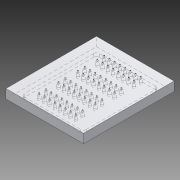
# Autodesk Inventor part: UNLHEP-14-01-P-001_ModuleChuck
Saved by Autodesk Inventor 2013 (Build 170138000, 138)
## iProperties
Created: 2014-01-06
Part Number: UNLHEP-14-01-P-001_ModuleChuck
Material: Aluminium 6061
Document SubType Name: Modeling
Designer: Frank Meier
Density: 2.71 g/cm^3
Project: UNL Pixel Phase I
Description: ModuleChuck
Mass: 472.689 g
Surface Area: 484.697 cm^2
Volume: 174.424 cm^3
Author: Frank Meier
Revision Number: 00
Title: Bonder Chuck
Autodesk Inventor part; units mm, degrees
ref_plane "YZ Plane" through (0, 0, 0) normal (1, 0, 0) x (0, 1, 0)
ref_plane "XZ Plane" through (0, 0, 0) normal (0, 1, 0) x (-1, 0, 0)
ref_plane "XY Plane" through (0, 0, 0) normal (0, 0, 1) x (1, 0, 0)
sketch "Skizze1" plane through (0, 0, 0) normal (0, 0, 1) x (1, 0, 0)
  line L0 (60, -70) -> (-60, -70)
  line L1 (-60, -70) -> (-60, 70)
  line L2 (-60, 70) -> (60, 70)
  line L3 (60, 70) -> (60, -70)
  line L4 (60, -70) -> (-60, 70) construction
  line L5 (-60, -70) -> (60, 70) construction
  point P0 (0, 0)
  dimension "d0" = 120
  dimension "d3" = 140
  constraints: 12 end point, 2 midpoint, 2 parallel, 1 horizontal, 1 perpendicular
  measures "d0" distance of L1.end L2.end
  measures "d3" distance of L0.end L1.end
extrude "Extrusion1" add sketch "Skizze1" along normal blind 14
sketch "Skizze2" plane through (0, 0, 0) normal (0, 0, -1) x (-1, 0, 0)
  line L0 (-32.4, 55.58) -> (32.4, 55.58) projected
  line L1 (32.4, 55.58) -> (32.4, 34.42) projected
  line L2 (32.4, 34.42) -> (-32.4, 34.42) projected
  line L3 (-32.4, 34.42) -> (-32.4, 55.58) projected
  point P0 (0, 0)
  point P1 (-28.35, 50.28)
  point P2 (-28.35, 39.72)
  point P3 (-20.25, 50.28)
  point P4 (-20.25, 39.72)
  point P5 (-12.15, 50.28)
  point P6 (-12.15, 39.72)
  point P7 (-4.05, 50.28)
  point P8 (-4.05, 39.72)
  point P9 (4.05, 50.28)
  point P10 (4.05, 39.72)
  point P11 (12.15, 50.28)
  point P12 (12.15, 39.72)
  point P13 (20.25, 50.28)
  point P14 (20.25, 39.72)
  point P15 (28.35, 50.28)
  point P16 (28.35, 39.72)
  dimension "d6" = 4.05
  dimension "d7" = 4.05
  dimension "d8" = 5.3
  dimension "d9" = 5.3
  dimension "d10" = 10.56
  dimension "d13" = 8.1
  constraints: 1 horizontal, 14 other
  measures "d6" distance from line of L3 point (-28.35, 50.28)
  measures "d7" distance from line of L3 point (-28.35, 39.72)
  measures "d8" distance from line of L0 point (-28.35, 50.28)
  measures "d9" distance from line of L2 point (-28.35, 39.72)
  measures "d10" distance of point (-28.35, 50.28) point (-28.35, 39.72)
  measures "d13" distance of point (-28.35, 50.28) point (-20.25, 50.28)
hole "Bohrung1" at (28.35, 50.28, 0) at (28.35, 39.72, 0) at (20.25, 50.28, 0) at (20.25, 39.72, 0) at (12.15, 50.28, 0) at (12.15, 39.72, 0) at (4.05, 50.28, 0) at (4.05, 39.72, 0) at (-4.05, 50.28, 0) at (-4.05, 39.72, 0) at (-12.15, 50.28, 0) at (-12.15, 39.72, 0) at (-20.25, 50.28, 0) at (-20.25, 39.72, 0) at (-28.35, 50.28, 0) at (-28.35, 39.72, 0) direction (0, 0, 1) diameter 1.5 end through all counterbore diameter 4 counterbore depth 11
pattern_linear "Rechteckige Anordnung1" count 4 spacing 30 along (0, -1, 0) of "Bohrung1"
sketch "Skizze3" plane through (0, 0, 0) normal (0, 0, -1) x (-1, 0, 0)
  circle A0 centre (28.35, -39.72) radius 2 projected
  circle A1 centre (28.35, -50.28) radius 2 projected
  circle A2 centre (20.25, -50.28) radius 2 projected
  circle A3 centre (12.15, -50.28) radius 2 projected
  circle A4 centre (4.05, -50.28) radius 2 projected
  circle A5 centre (-4.05, -50.28) radius 2 projected
  circle A6 centre (-12.15, -50.28) radius 2 projected
  circle A7 centre (-20.25, -50.28) radius 2 projected
  circle A8 centre (-28.35, -50.28) radius 2 projected
  circle A9 centre (-28.35, -39.72) radius 2 projected
  circle A10 centre (-20.25, -39.72) radius 2 projected
  circle A11 centre (-12.15, -39.72) radius 2 projected
  circle A12 centre (-4.05, -39.72) radius 2 projected
  circle A13 centre (4.05, -39.72) radius 2 projected
  circle A14 centre (12.15, -39.72) radius 2 projected
  circle A15 centre (20.25, -39.72) radius 2 projected
  circle A16 centre (28.35, -9.72) radius 2 projected
  circle A17 centre (28.35, -20.28) radius 2 projected
  circle A18 centre (20.25, -20.28) radius 2 projected
  circle A19 centre (12.15, -20.28) radius 2 projected
  circle A20 centre (4.05, -20.28) radius 2 projected
  circle A21 centre (-4.05, -20.28) radius 2 projected
  circle A22 centre (-12.15, -20.28) radius 2 projected
  circle A23 centre (-20.25, -20.28) radius 2 projected
  circle A24 centre (-28.35, -20.28) radius 2 projected
  circle A25 centre (-28.35, -9.72) radius 2 projected
  circle A26 centre (-20.25, -9.72) radius 2 projected
  circle A27 centre (-12.15, -9.72) radius 2 projected
  circle A28 centre (-4.05, -9.72) radius 2 projected
  circle A29 centre (4.05, -9.72) radius 2 projected
  circle A30 centre (12.15, -9.72) radius 2 projected
  circle A31 centre (20.25, -9.72) radius 2 projected
  circle A32 centre (28.35, 20.28) radius 2 projected
  circle A33 centre (28.35, 9.72) radius 2 projected
  circle A34 centre (20.25, 9.72) radius 2 projected
  circle A35 centre (12.15, 9.72) radius 2 projected
  circle A36 centre (4.05, 9.72) radius 2 projected
  circle A37 centre (-4.05, 9.72) radius 2 projected
  circle A38 centre (-12.15, 9.72) radius 2 projected
  circle A39 centre (-20.25, 9.72) radius 2 projected
  circle A40 centre (-28.35, 9.72) radius 2 projected
  circle A41 centre (-28.35, 20.28) radius 2 projected
  circle A42 centre (-20.25, 20.28) radius 2 projected
  circle A43 centre (-12.15, 20.28) radius 2 projected
  circle A44 centre (-4.05, 20.28) radius 2 projected
  circle A45 centre (4.05, 20.28) radius 2 projected
  circle A46 centre (12.15, 20.28) radius 2 projected
  circle A47 centre (20.25, 20.28) radius 2 projected
  circle A48 centre (28.35, 50.28) radius 2 projected
  circle A49 centre (20.25, 50.28) radius 2 projected
  circle A50 centre (12.15, 50.28) radius 2 projected
  circle A51 centre (4.05, 50.28) radius 2 projected
  circle A52 centre (-4.05, 50.28) radius 2 projected
  circle A53 centre (-12.15, 50.28) radius 2 projected
  circle A54 centre (-20.25, 50.28) radius 2 projected
  circle A55 centre (-28.35, 50.28) radius 2 projected
  circle A56 centre (-28.35, 39.72) radius 2 projected
  circle A57 centre (-20.25, 39.72) radius 2 projected
  circle A58 centre (-12.15, 39.72) radius 2 projected
  circle A59 centre (-4.05, 39.72) radius 2 projected
  circle A60 centre (4.05, 39.72) radius 2 projected
  circle A61 centre (12.15, 39.72) radius 2 projected
  circle A62 centre (20.25, 39.72) radius 2 projected
  circle A63 centre (28.35, 39.72) radius 2 projected
  line L0 (-60, -70) -> (60, -70) projected
  line L1 (60, -70) -> (60, 70) projected
  line L2 (60, 70) -> (-60, 70) projected
  line L3 (-60, 70) -> (-60, -70) projected
  line L4 (-48, 58) -> (48, 58)
  line L5 (48, 58) -> (48, -58)
  line L6 (48, -58) -> (-48, -58)
  line L7 (-48, -58) -> (-48, 58)
  point P0 (0, 0)
  dimension "d28" = 12
  constraints: 8 end point, 3 other
  measures "d28" distance between parallel lines of L3 L7
extrude "Extrusion2" cut sketch "Skizze3" against normal blind 5 contours L4 L5 L6 L7
fillet "Rundung1" radius 4 4 edges at (48, 58, 2.5) (48, -58, 2.5) (-48, 58, 2.5) (-48, -58, 2.5)
